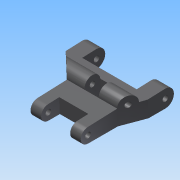
# Autodesk Inventor part: Transmission Plate - Top
Saved by Autodesk Inventor 2014 (Build 180170000, 170)
## iProperties
Created: 2011-09-21
Part Number: Transmission Plate - Top
Document SubType Name: Modeling
Designer: dgitz
Density: 1 g/cm^3
Material: Generic
Appearance: Smooth - Medium Gray
d5: 0.115 in
d8: 1.800 in
d9: 0.00 deg
d21: 1.280 in
d22: 0.180 in
d24: 0.00 deg
d26: 1.300 in
d27: 0.230 in
d28: 0.230 in
d29: 0.400 in
d31: 0.490 in
d32: 0.310 in
d33: 0.310 in
d34: 0.400 in
d36: 1.180 in
d37: 0.630 in
d38: 0.120 in
d39: 0.157 in
d40: 0.188 in
d41: 1.375 in
d42: 0.530 in
d43: 0.340 in
d44: 0.354 in
d45: 0.301 in
Author: dgitz
Autodesk Inventor part; units mm, degrees
sketch "Sketch3" plane through (0, 0, 0) normal (1, 0, 0) x (0, 1, 0)
  arc A0 (-1.1214, 20.6041) -> (-9.0936, 20.4414) centre (-5.1058, 20.4414) ccw
  circle A1 centre (-5.1058, 20.4414) radius 1.524
  arc A2 (-9.0936, -17.5316) -> (0.4274, -17.3373) centre (-4.3311, -17.5316) ccw
  circle A3 centre (-4.3311, -17.5316) radius 1.524
  arc A4 (-0.102, -4.3672) -> (-0.4576, 4.3443) centre (0, 0) ccw
  circle A5 centre (0, 0) radius 1.4605
  line L0 (-9.0936, 20.4414) -> (-9.0936, -17.5316)
  line L1 (-1.1214, 20.6041) -> (-0.4576, 4.3443)
  line L2 (-0.102, -4.3672) -> (0.4274, -17.3373)
  line L3 (0, 0) -> (0, 35.9976) construction
  line L4 (0, 0) -> (20.0348, 0) construction
  line L5 (9.2339, 18.9174) -> (-10.5183, 18.9174) construction
  line L6 (11.5384, -16.0076) -> (-16.1147, -16.0076) construction
  line L7 (4.3684, 5.3055) -> (4.3684, -5.6899) construction
  line L8 (-1.4605, 3.5835) -> (-1.4605, -5.6899) construction
  dimension "d5" = 2.921
  dimension "d38" = 3.048
  dimension "d39" = 3.9878
  dimension "d40" = 4.7625
  dimension "d41" = 34.925
  dimension "d42" = 13.462
  dimension "d43" = 8.636
  dimension "d44" = 8.9916
  dimension "d45" = 7.6331
  constraints: 18 end point, 10 tangent, 6 centre point, 6 point on circle, 5 coincident, 3 parallel, 2 perpendicular, 1 equal radius, 1 vertical
  measures "d5" diameter of A5
  measures "d38" diameter of A1
  measures "d39" radius of A0
  measures "d40" radius of A2
  measures "d41" distance between parallel lines of L6 L5
  measures "d42" distance between parallel lines of L0 L7
  measures "d43" distance from line of L0 L1.end
  measures "d44" distance from line of L0 L2.start
  measures "d45" distance between parallel lines of L0 L8
extrude "Extrusion1" add sketch "Sketch3" along normal mid plane 45.72
ref_plane "Work Plane1" through (0, 4.3647, 0.1782) normal (0, 0.9991679, 0.0407857) x (-1, 0, 0)
sketch "Sketch5" plane through (0, 4.3647, 0.1782) normal (0, 0.9991679, 0.0407857) x (-1, 0, 0)
  line L0 (-22.86, -7.8915) -> (-22.86, 24.6205)
  line L1 (-22.86, 24.6205) -> (-18.288, 24.6205)
  line L2 (-18.288, 24.6205) -> (-18.288, 4.3594)
  line L3 (-18.288, 4.3594) -> (-22.86, -7.8915)
  line L4 (-22.86, 20.6327) -> (-22.86, 4.3594) projected
  line L5 (22.86, 0) -> (-22.86, 0) projected
  line L6 (22.86, 24.6205) -> (-22.86, 24.6205) projected
  line L7 (22.86, 4.3594) -> (-22.86, 4.3594) projected
  line L8 (-22.86, 4.3594) -> (-22.86, -4.3594) projected
  line L9 (22.86, -4.3594) -> (-22.86, -4.3594) projected
  line L10 (22.86, -4.3594) -> (22.86, 4.3594) projected
  line L11 (22.86, 4.3594) -> (-22.86, 4.3594) projected
  line L12 (22.86, 24.6205) -> (22.86, -8.3995)
  line L13 (22.86, -8.3995) -> (9.398, 4.3594)
  line L14 (9.398, 4.3594) -> (9.398, 24.6205)
  line L15 (22.86, -22.1028) -> (-22.86, -22.1028) projected
  line L16 (14.986, -9.6568) -> (-14.986, -9.6568)
  line L17 (-14.986, -9.6568) -> (-14.986, -22.1028)
  line L18 (-14.986, -22.1028) -> (14.986, -22.1028)
  line L19 (14.986, -22.1028) -> (14.986, -9.6568)
  line L20 (3.556, 14.4605) -> (-12.446, 14.4605)
  line L21 (-12.446, 14.4605) -> (-12.446, 24.6205)
  line L22 (-12.446, 24.6205) -> (3.556, 24.6205)
  line L23 (3.556, 24.6205) -> (3.556, 14.4605)
  line L24 (-22.86, -4.3594) -> (-22.86, -17.3403) projected
  line L25 (22.86, -17.3403) -> (22.86, -4.3594) projected
  line L26 (-8.128, 4.3594) -> (-0.254, 4.3594)
  line L27 (-0.254, 4.3594) -> (-0.254, -4.3594)
  line L28 (-0.254, -4.3594) -> (-8.128, -4.3594)
  line L29 (-8.128, -4.3594) -> (-8.128, 4.3594)
  point P0 (0, 0)
  dimension "d21" = 32.512
  dimension "d22" = 4.572
  dimension "d26" = 33.02
  dimension "d27" = 5.842
  dimension "d28" = 5.842
  dimension "d29" = 10.16
  dimension "d31" = 12.446
  dimension "d32" = 7.874
  dimension "d33" = 7.874
  dimension "d34" = 10.16
  dimension "d36" = 29.972
  dimension "d37" = 16.002
  constraints: 38 end point, 10 point on line, 7 parallel, 4 perpendicular, 3 horizontal, 2 vertical
  measures "d21" distance from line of L0.start L1
  measures "d22" distance between parallel lines of L0 L2
  measures "d26" distance from line of L6 L12.end
  measures "d27" distance between parallel lines of L14 L23
  measures "d28" distance between parallel lines of L2 L21
  measures "d29" distance between parallel lines of L6 L20
  measures "d31" distance between parallel lines of L16 L18
  measures "d32" distance between parallel lines of L25 L19
  measures "d33" distance between parallel lines of L27 L29
  measures "d34" distance between parallel lines of L29 L2
  measures "d36" distance between parallel lines of L17 L19
  measures "d37" distance between parallel lines of L23 L21
extrude "Extrusion2" cut sketch "Sketch5" against normal up to surface contours L0 L9 L3 | L0 L5 L3 L9 | L0 L7 L3 L5 | L29 L5 L27 L9 | L0 L1 L2 L7 | L29 L7 L27 L5 | L13 L5 L10 L9 | L9 L12 L13 | L6 L23 L20 L21 | L13 L7 L10 L5 | L14 L6 L12 L7 | L15 L17 L16 L19 surface through (0, -9.0936, -17.5316) normal (0, -1, 0)
ref_plane "Work Plane2" through (0, -5.1058, 24.4292) normal (0, 0, 1) x (1, 0, 0)
ref_plane "Work Plane3" through (0, -4.3311, -22.2941) normal (0, 0, 1) x (1, 0, 0)
body "Solid1"
